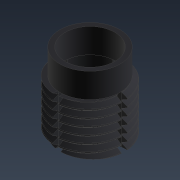
# Autodesk Inventor part: bottomPiece2
Saved by Autodesk Inventor 2022 (Build 260153000, 153)
## iProperties
Created: 2022-07-02
Part Number: bottomPiece2
Material: Generic
Document SubType Name: Modeling
Designer: User
Density: 1 g/cm^3
Appearance: Default
Author: User
## iProperties of the stored document bottomPiece_3DPrint.ipt
Created: 2022-07-04
Part Number: bottomPiece_3DPrint
Material: Generic
Document SubType Name: Modeling
Designer: User
Density: 1 g/cm^3
Appearance: Default
Author: User
Autodesk Inventor part; units mm, degrees
ref_plane "YZ Plane" through (0, 0, 0) normal (1, 0, 0) x (0, 1, 0)
ref_plane "XZ Plane" through (0, 0, 0) normal (0, 1, 0) x (-1, 0, 0)
ref_plane "XY Plane" through (0, 0, 0) normal (0, 0, 1) x (1, 0, 0)
sketch "Sketch1" plane through (0, 0, 0) normal (0, 1, 0) x (-1, 0, 0)
  circle A0 centre (0, 0) radius 10.1
  circle A1 centre (0, 0) radius 14.1
  dimension "d0" = 20.2
  dimension "d1" = 28.2
  constraints: 2 centre point, 2 coincident
  measures "d0" diameter of A0
  measures "d1" diameter of A1
extrude "Extrusion1" add sketch "Sketch1" along normal blind 20
chamfer "Chamfer1" [suppressed]
sketch "Sketch12" plane through (0, 0, 0) normal (0, -1, 0) x (1, 0, 0)
  circle A0 centre (0, 0) radius 10.1 projected
  circle A1 centre (0, 0) radius 10.2
  circle A2 centre (0, 0) radius 12.2
  dimension "d74" = 20.4
  dimension "d139" = 24.4
  constraints: 2 centre point, 2 coincident
  measures "d74" diameter of A1
  measures "d139" diameter of A2
extrude "Extrusion3" add sketch "Sketch12" along normal blind 10 contours A2
thread "M22x3" size "M22x3" class "6g" standard "ANSI Metric M Profile" full length
sketch "Sketch29" plane through (0, 20, 0) normal (1, 0, 0) x (0, 0, 1)
  line L0 (14.1, 0) -> (14.1, 20)
  line L1 (14.1, 20) -> (11.8756, 20)
  line L2 (11.8756, 20) -> (11.8756, 0)
  line L3 (11.8756, 0) -> (14.1, 0)
  line L4 (0, -9.9256) -> (0, 36.6543) projected
  constraints: 8 end point
revolve "Revolution16" cut sketch "Sketch29" angle 360 about axis through (0, 20, 0) along (0, -1, 0)
sketch "Sketch30" plane through (0, 20, 0) normal (1, 0, 0) x (0, 0, 1)
  line L0 (14.1, 0) -> (14.1, 20)
  line L1 (14.1, 20) -> (11.8756, 20)
  line L2 (11.8756, 20) -> (11.8756, 0)
  line L3 (11.8756, 0) -> (14.1, 0)
  line L4 (0, -9.9256) -> (0, 36.6543) projected
  constraints: 8 end point
revolve "Revolution17" add sketch "Sketch30" angle 360 about axis through (0, 20, 0) along (0, -1, 0) separate body
sketch "Sketch28" plane through (0, 20, 0) normal (-1, 0, 0) x (0, -1, 0)
  line L0 (-1.7501, -12.0275) -> (-1.5001, -12.0275) construction
  line L1 (0.2499, -13.9485) -> (-0.0001, -14.4287) construction
  line L2 (-3.0001, -14.4287) -> (-3.2501, -13.9485) construction
  line L3 (-1.2501, -12.0275) -> (-1.5001, -11.5472) construction
  line L4 (-1.5001, -11.5472) -> (-1.7501, -12.0275) construction
  line L5 (-3.0001, -14.4287) -> (-2.7501, -13.9485) construction
  line L6 (-1.2501, -12.0275) -> (-0.2501, -13.9485)
  line L7 (-3.2501, -13.9485) -> (-2.7501, -13.9485) construction
  arc A0 (-3.2501, -13.9485) -> (-3.0001, -14.1002) centre (-3.0001, -13.8183) ccw construction
  line L8 (0.2499, -13.9485) -> (-0.2501, -13.9485) construction
  line L9 (-3.0001, -14.4287) -> (-3.0001, -13.9485) construction
  line L10 (-0.0001, -14.4287) -> (-0.0001, -13.9485) construction
  line L11 (-1.5001, -11.5472) -> (-1.5001, -11.8758) construction
  line L12 (-3.0001, -14.1002) -> (-0.0001, -14.1002)
  arc A1 (-3.0001, -14.1002) -> (-2.7501, -13.9485) centre (-3.0001, -13.8183) ccw
  line L13 (-0.2501, -13.9485) -> (-0.0001, -14.4287) construction
  line L14 (-2.7501, -13.9485) -> (-1.7501, -12.0275)
  line L15 (-0.0001, -0.0002) -> (-0.0001, 0.0177)
  line L16 (-0.0001, 0.0177) -> (-0.0001, -0.0002)
  line L17 (-0.0001, -0.0002) -> (0.0334, -0.0002)
  arc A2 (-0.2501, -13.9485) -> (-0.0001, -14.1002) centre (-0.0001, -13.8183) ccw
  arc A3 (-0.0001, -14.1002) -> (0.2499, -13.9485) centre (-0.0001, -13.8183) ccw construction
  arc A4 (-1.5001, -11.8758) -> (-1.7501, -12.0275) centre (-1.5001, -12.1576) ccw
  arc A5 (-1.2501, -12.0275) -> (-1.5001, -11.8758) centre (-1.5001, -12.1576) ccw
  line L18 (-1.5001, -11.8758) -> (-1.5001, -12.0275) construction
  line L19 (-1.5001, -12.0275) -> (-1.2501, -12.0275) construction
  dimension "d163" = 55
  dimension "d164" = 0.4803
  dimension "d165" = 0.4803
  dimension "Sketch28_ThreadOffset" = 0
  dimension "Sketch28_MajorRadius" = 14.1
  dimension "d168" = 3
  dimension "Sketch28_MinorRadius" = 11.8756
  constraints: 40 end point, 12 point on circle, 10 parallel, 8 tangent, 6 centre point, 6 collinear, 2 midpoint, 2 point on line, 1 horizontal, 1 perpendicular, 3 other
  measures "d163" angle of L6 L14
  measures "d164" distance of L3.end L0.end
  measures "d165" distance of L1.end L10.end
  measures "Sketch28_ThreadOffset" distance between parallel lines of L15 L10
  measures "Sketch28_MajorRadius" distance from line of L12 L15.start
  measures "d168" distance from line of L1.end L9
  measures "Sketch28_MinorRadius" distance edge to line of A5 L17
coil "Coil8" sketch "Sketch28" operation cut axis through (0, 20, 0) along (0, -1, 0) pitch 3.003 turns 8.658009 hand right bodies 2
sketch "Sketch31" plane through (0, 0, 0) normal (1, 0, 0) x (0, 1, 0)
  line L0 (0, 10.2) -> (0, -10.2) projected
  line L1 (0, -10.2) -> (20, -10.1)
  line L2 (20, -10.1) -> (0, -10.1) projected
  line L3 (0, 0) -> (7.1062, 0) construction
  constraints: 4 end point, 1 point on line
revolve "Revolution18" cut sketch "Sketch31" angle 360 about axis through (0, 0, 0) along (0, 1, 0) bodies 1
sketch "Sketch8" plane through (0, 0, 0) normal (0, 1, 0) x (-1, 0, 0)
  circle A0 centre (0, 0) radius 14.1
  line L0 (0, 0) -> (14.0463, -1.2289)
  line L1 (0, 0) -> (14.1, 0) construction
  line L2 (0, 0) -> (14.0463, 1.2289)
  line L3 (0, 0) -> (-14.0463, -1.2289)
  line L4 (0, 0) -> (-14.0463, 1.2289)
  line L5 (0, 0) -> (1.2289, 14.0463)
  line L6 (0, 0) -> (-1.2289, 14.0463)
  line L7 (0, 3.6676) -> (0, -3.2664) construction
  line L8 (0, 0) -> (1.2289, -14.0463)
  line L9 (0, 0) -> (-1.2289, -14.0463)
  dimension "d46" = 28.2
  dimension "d47" = 5
  dimension "d183" = 10
  constraints: 20 end point, 5 point on circle, 4 collinear, 1 centre point, 1 coincident, 1 equal length, 1 horizontal, 1 symmetric about line, 1 vertical, 1 other
  measures "d46" diameter of A0
  measures "d47" angle of L0 L1
  measures "d183" angle of L6 L5
extrude "slot" cut sketch "Sketch8" along normal through all contours A0 L0 L2 | L5 L6 A0 | L3 A0 L4 | L8 A0 L9 bodies 1 2
sketch "Sketch24" plane through (0, 15, 0) normal (0, -1, 0) x (1, 0, 0)
  circle A0 centre (0, 0) radius 14
  circle A1 centre (0, 0) radius 14.1
  point P0 (-13.8648, -1.9407)
  point P1 (13.6079, 3.2903)
  point P2 (13.8648, 1.9407)
  point P3 (13.8661, -1.9318)
  dimension "d141" = 28.2
  constraints: 2 centre point, 2 coincident, 3 other
  measures "d141" diameter of A1
equation "\"d163\" = d170"
equation "\"d164\" = 0.160083 * Sketch28_Pitch"
equation "\"d165\" = 0.160083 * Sketch28_Pitch"
equation "\"d168\" = Sketch28_Pitch"
equation "\"d46\" = d1"
equation "\"d183\" = 2 * d47"
equation "\"d13\" = 55deg"
equation "\"Sketch2_Pitch\" = 1.5"
equation "\"d34\" = 55deg"
equation "\"Sketch5_Pitch\" = 2"
equation "\"d60\" = 55deg"
equation "\"Sketch9_Pitch\" = 2"
equation "\"d83\" = 55deg"
equation "\"Sketch14_Pitch\" = 2"
equation "\"d104\" = 55deg"
equation "\"Sketch17_Pitch\" = 3"
equation "\"d125\" = 55deg"
equation "\"Sketch20_Pitch\" = 3"
equation "\"d151\" = 55deg"
equation "\"Sketch25_Pitch\" = 3"
equation "\"d170\" = 55deg"
equation "\"Sketch28_Pitch\" = 3"
body "Solid1"
body "Solid9"
